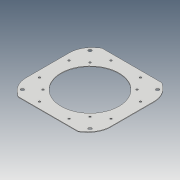
# Autodesk Inventor part: 모터드라이버 지지대 철판가공
Saved by Autodesk Inventor 2018 (Build 220112000, 112)
## iProperties
Created: 2018-10-26
Part Number: 모터드라이버 지지대 철판가공
Material: 일반
Document SubType Name: Modeling
Designer: dhksr
Density: 1 g/cm^3
Appearance: 기본값
Author: dhksr
Autodesk Inventor part; units mm, degrees
ref_plane "YZ Plane" through (0, 0, 0) normal (1, 0, 0) x (0, 1, 0)
ref_plane "XZ Plane" through (0, 0, 0) normal (0, 1, 0) x (-1, 0, 0)
ref_plane "XY Plane" through (0, 0, 0) normal (0, 0, 1) x (1, 0, 0)
sketch "스케치1" plane through (0, 0, 0) normal (0, 0, 1) x (1, 0, 0)
  circle A0 centre (0, 0) radius 60 construction
  line L0 (0, 0) -> (0, 95.3997)
  line L1 (0, 0) -> (-132.5472, 0)
  line L2 (52.5, 52.5) -> (-52.5, 52.5)
  line L3 (-52.5, 52.5) -> (-52.5, -52.5)
  line L4 (-52.5, -52.5) -> (52.5, -52.5)
  line L5 (52.5, -52.5) -> (52.5, 52.5)
  line L6 (52.5, 52.5) -> (-52.5, -52.5) construction
  line L7 (-52.5, 52.5) -> (52.5, -52.5) construction
  arc A1 (-46.6369, 65) -> (-46.6369, -65) centre (0, 0) ccw
  arc A2 (46.6369, -65) -> (46.6369, 65) centre (0, 0) ccw
  line L8 (-46.6369, 65) -> (46.6369, 65)
  line L9 (-46.6369, -65) -> (46.6369, -65)
  line L10 (0, 0) -> (104.7447, 43.3867)
  line L11 (0, 0) -> (113.3748, 0) construction
  circle A3 centre (55.4328, 22.961) radius 1.5
  dimension "d0" = 120
  dimension "d49" = 105
  dimension "d50" = 105
  dimension "d56" = 22.5
  dimension "d57" = 3
  constraints: 24 end point, 5 horizontal, 4 midpoint, 4 point on circle, 3 centre point, 2 coincident, 2 parallel, 1 equal length, 1 perpendicular, 1 point on line, 1 vertical, 3 other
  measures "d49" distance of L4.end L3.end
  measures "d50" distance of L3.end L2.end
  measures "d56" angle of L11 L10
  measures "d57" diameter of A3
extrude "돌출1" add sketch "스케치1" along normal blind 1
sketch "스케치5" plane through (0, 0, 1) normal (0, 0, 1) x (1, 0, 0)
  arc A0 (46.6369, -65) -> (46.6369, 65) centre (0, 0) ccw projected
  circle A1 centre (55.4328, 22.961) radius 1.5 projected
  circle A2 centre (55.4328, 22.961) radius 1.5
  circle A3 centre (22.961, 55.4328) radius 1.5
  circle A4 centre (-22.961, 55.4328) radius 1.5
  circle A5 centre (-55.4328, 22.961) radius 1.5
  circle A6 centre (-55.4328, -22.961) radius 1.5
  circle A7 centre (-22.961, -55.4328) radius 1.5
  circle A8 centre (22.961, -55.4328) radius 1.5
  circle A9 centre (55.4328, -22.961) radius 1.5
  dimension "d60" = 360
  constraints: 8 centre point, 1 coincident, 1 concentric, 17 other
extrude "돌출5" cut sketch "스케치5" against normal through all
sketch "스케치6" plane through (0, 0, 1) normal (0, 0, 1) x (1, 0, 0)
  arc A0 (-46.6369, 65) -> (-46.6369, -65) centre (0, 0) ccw projected
  line L0 (36.5, 36.5) -> (-36.5, 36.5) construction
  line L1 (-36.5, 36.5) -> (-36.5, -36.5) construction
  line L2 (-36.5, -36.5) -> (36.5, -36.5) construction
  line L3 (36.5, -36.5) -> (36.5, 36.5) construction
  line L4 (36.5, 36.5) -> (-36.5, -36.5) construction
  line L5 (-36.5, 36.5) -> (36.5, -36.5) construction
  circle A1 centre (-36.5, 36.5) radius 1.5
  dimension "d64" = 73
  dimension "d65" = 73
  dimension "d66" = 3
  constraints: 12 end point, 2 midpoint, 2 parallel, 1 centre point, 1 coincident, 1 horizontal, 1 perpendicular
  measures "d64" distance of L2.end L1.end
  measures "d65" distance of L1.end L0.end
  measures "d66" diameter of A1
extrude "돌출6" cut sketch "스케치6" against normal through all
pattern_circular "원형 패턴1" count 4 over 360 about axis through (0, 0, 0) along (0, 0, 1) of "돌출6"
sketch "스케치7" plane through (0, 0, 1) normal (0, 0, 1) x (1, 0, 0)
  arc A0 (-46.6369, 65) -> (-46.6369, -65) centre (0, 0) ccw projected
  line L0 (52.5, 52.5) -> (-52.5, 52.5) construction
  line L1 (-52.5, 52.5) -> (-52.5, -52.5) construction
  line L2 (-52.5, -52.5) -> (52.5, -52.5) construction
  line L3 (52.5, -52.5) -> (52.5, 52.5) construction
  line L4 (52.5, 52.5) -> (-52.5, -52.5) construction
  line L5 (-52.5, 52.5) -> (52.5, -52.5) construction
  circle A1 centre (-52.5, 52.5) radius 2.5
  dimension "d72" = 105
  dimension "d73" = 105
  dimension "d74" = 5
  constraints: 12 end point, 2 midpoint, 2 parallel, 1 centre point, 1 coincident, 1 horizontal, 1 perpendicular
  measures "d72" distance of L2.end L1.end
  measures "d73" distance of L1.end L0.end
  measures "d74" diameter of A1
extrude "돌출7" cut sketch "스케치7" against normal through all
pattern_circular "원형 패턴2" count 4 over 360 about axis through (0, 0, 0) along (0, 0, 1) of "돌출7"
sketch "스케치9" plane through (0, 0, 1) normal (0, 0, 1) x (1, 0, 0)
  arc A0 (-46.6369, 65) -> (-46.6369, -65) centre (0, 0) ccw projected
  line L0 (-34.8236, -59) -> (-59, -34.8236) projected
  line L1 (-59, -34.8236) -> (-59, 34.8236) projected
  line L2 (-59, 34.8236) -> (-34.8236, 59) projected
  line L3 (-34.8236, 59) -> (34.8236, 59) projected
  line L4 (34.8236, 59) -> (59, 34.8236) projected
  line L5 (59, 34.8236) -> (59, -34.8236) projected
  line L6 (59, -34.8236) -> (34.8236, -59) projected
  line L7 (34.8236, -59) -> (-34.8236, -59) projected
  circle A1 centre (52.5, -52.5) radius 2.5 projected
  circle A2 centre (-52.5, 52.5) radius 2.5 projected
  circle A3 centre (-52.5, -52.5) radius 2.5 projected
  circle A4 centre (52.5, 52.5) radius 2.5 projected
  line L8 (-84.5, -70.75) -> (65.5, -70.75) projected
  line L9 (65.5, -70.75) -> (65.5, 70.75) projected
  line L10 (65.5, 70.75) -> (-84.5, 70.75) projected
  line L11 (-84.5, 70.75) -> (-84.5, -70.75) projected
  circle A5 centre (0, 0) radius 45
  dimension "d80" = 90
  constraints: 1 centre point, 1 coincident
  measures "d80" diameter of A5
extrude "돌출8" cut sketch "스케치9" against normal through all contours A5
sketch "스케치11" plane through (0, 0, 1) normal (0, 0, 1) x (1, 0, 0)
  line L0 (65.5, -70.75) -> (65.5, 70.75) projected
  line L1 (65.5, 70.75) -> (105.9964, 70.75)
  line L2 (105.9964, 70.75) -> (105.9964, -90.2742)
  line L3 (105.9964, -90.2742) -> (65.5, -90.2742)
  line L4 (65.5, -90.2742) -> (65.5, 70.75)
  constraints: 8 end point, 2 parallel, 1 horizontal, 1 perpendicular
extrude "돌출9" cut sketch "스케치11" against normal through all
mirror "미러3" about plane through (0, 0, 0) normal (1, 0, 0) of "돌출9"
fillet "모깎기3" radius 33.75 4 edges at (65.5, 45.932, 0.5) (65.5, -45.932, 0.5) (-65.5, -45.932, 0.5) (-65.5, 45.932, 0.5)
